Autodesk Inventor part; units mm, degrees
(part 3 of 4)
  circle A565 centre (25.95, -42.62) radius 1.125 construction
  circle A566 centre (31.03, -42.62) radius 1.125 construction
  circle A567 centre (36.11, -42.62) radius 1.125 construction
  circle A568 centre (41.19, -42.62) radius 1.125 construction
  circle A569 centre (46.27, -42.62) radius 1.125 construction
  circle A570 centre (51.35, -42.62) radius 1.125 construction
  circle A571 centre (56.43, -42.62) radius 1.125 construction
  circle A572 centre (61.51, -42.62) radius 1.125 construction
  circle A573 centre (66.59, -42.62) radius 1.125 construction
  circle A574 centre (71.67, -42.62) radius 1.125 construction
  circle A575 centre (76.75, -42.62) radius 1.125 construction
  circle A576 centre (81.83, -42.62) radius 1.125 construction
  circle A577 centre (10.71, -40.08) radius 1.125 construction
  circle A578 centre (15.79, -40.08) radius 1.125 construction
  circle A579 centre (20.87, -40.08) radius 1.125 construction
  circle A580 centre (25.95, -40.08) radius 1.125 construction
  circle A581 centre (31.03, -40.08) radius 1.125 construction
  circle A582 centre (36.11, -40.08) radius 1.125 construction
  circle A583 centre (41.19, -40.08) radius 1.125 construction
  circle A584 centre (46.27, -40.08) radius 1.125 construction
  circle A585 centre (51.35, -40.08) radius 1.125 construction
  circle A586 centre (56.43, -40.08) radius 1.125 construction
  circle A587 centre (61.51, -40.08) radius 1.125 construction
  circle A588 centre (66.59, -40.08) radius 1.125 construction
  circle A589 centre (71.67, -40.08) radius 1.125 construction
  circle A590 centre (76.75, -40.08) radius 1.125 construction
  circle A591 centre (81.83, -40.08) radius 1.125 construction
  circle A592 centre (10.71, -37.54) radius 1.125 construction
  circle A593 centre (15.79, -37.54) radius 1.125 construction
  circle A594 centre (20.87, -37.54) radius 1.125 construction
  circle A595 centre (25.95, -37.54) radius 1.125 construction
  circle A596 centre (31.03, -37.54) radius 1.125 construction
  circle A597 centre (36.11, -37.54) radius 1.125 construction
  circle A598 centre (41.19, -37.54) radius 1.125 construction
  circle A599 centre (46.27, -37.54) radius 1.125 construction
  circle A600 centre (51.35, -37.54) radius 1.125 construction
  circle A601 centre (56.43, -37.54) radius 1.125 construction
  circle A602 centre (61.51, -37.54) radius 1.125 construction
  circle A603 centre (66.59, -37.54) radius 1.125 construction
  circle A604 centre (71.67, -37.54) radius 1.125 construction
  circle A605 centre (76.75, -37.54) radius 1.125 construction
  circle A606 centre (81.83, -37.54) radius 1.125 construction
  circle A607 centre (10.71, -35) radius 1.125 construction
  circle A608 centre (15.79, -35) radius 1.125 construction
  circle A609 centre (20.87, -35) radius 1.125 construction
  circle A610 centre (25.95, -35) radius 1.125 construction
  circle A611 centre (31.03, -35) radius 1.125 construction
  circle A612 centre (36.11, -35) radius 1.125 construction
  circle A613 centre (41.19, -35) radius 1.125 construction
  circle A614 centre (46.27, -35) radius 1.125 construction
  circle A615 centre (51.35, -35) radius 1.125 construction
  circle A616 centre (56.43, -35) radius 1.125 construction
  circle A617 centre (61.51, -35) radius 1.125 construction
  circle A618 centre (66.59, -35) radius 1.125 construction
  circle A619 centre (71.67, -35) radius 1.125 construction
  circle A620 centre (76.75, -35) radius 1.125 construction
  circle A621 centre (81.83, -35) radius 1.125 construction
  circle A622 centre (10.71, -32.46) radius 1.125 construction
  circle A623 centre (15.79, -32.46) radius 1.125 construction
  circle A624 centre (20.87, -32.46) radius 1.125 construction
  circle A625 centre (25.95, -32.46) radius 1.125 construction
  circle A626 centre (31.03, -32.46) radius 1.125 construction
  circle A627 centre (36.11, -32.46) radius 1.125 construction
  circle A628 centre (41.19, -32.46) radius 1.125 construction
  circle A629 centre (46.27, -32.46) radius 1.125 construction
  circle A630 centre (51.35, -32.46) radius 1.125 construction
  circle A631 centre (56.43, -32.46) radius 1.125 construction
  circle A632 centre (61.51, -32.46) radius 1.125 construction
  circle A633 centre (66.59, -32.46) radius 1.125 construction
  circle A634 centre (71.67, -32.46) radius 1.125 construction
  circle A635 centre (76.75, -32.46) radius 1.125 construction
  circle A636 centre (81.83, -32.46) radius 1.125 construction
  circle A637 centre (10.71, -29.92) radius 1.125 construction
  circle A638 centre (15.79, -29.92) radius 1.125 construction
  circle A639 centre (20.87, -29.92) radius 1.125 construction
  circle A640 centre (25.95, -29.92) radius 1.125 construction
  circle A641 centre (31.03, -29.92) radius 1.125 construction
  circle A642 centre (36.11, -29.92) radius 1.125 construction
  circle A643 centre (41.19, -29.92) radius 1.125 construction
  circle A644 centre (46.27, -29.92) radius 1.125 construction
  circle A645 centre (51.35, -29.92) radius 1.125 construction
  circle A646 centre (56.43, -29.92) radius 1.125 construction
  circle A647 centre (61.51, -29.92) radius 1.125 construction
  circle A648 centre (66.59, -29.92) radius 1.125 construction
  circle A649 centre (71.67, -29.92) radius 1.125 construction
  circle A650 centre (76.75, -29.92) radius 1.125 construction
  circle A651 centre (81.83, -29.92) radius 1.125 construction
  circle A652 centre (10.71, -27.38) radius 1.125 construction
  circle A653 centre (15.79, -27.38) radius 1.125 construction
  circle A654 centre (20.87, -27.38) radius 1.125 construction
  circle A655 centre (25.95, -27.38) radius 1.125 construction
  circle A656 centre (31.03, -27.38) radius 1.125 construction
  circle A657 centre (36.11, -27.38) radius 1.125 construction
  circle A658 centre (41.19, -27.38) radius 1.125 construction
  circle A659 centre (46.27, -27.38) radius 1.125 construction
  circle A660 centre (51.35, -27.38) radius 1.125 construction
  circle A661 centre (56.43, -27.38) radius 1.125 construction
  circle A662 centre (61.51, -27.38) radius 1.125 construction
  circle A663 centre (66.59, -27.38) radius 1.125 construction
  circle A664 centre (71.67, -27.38) radius 1.125 construction
  circle A665 centre (76.75, -27.38) radius 1.125 construction
  circle A666 centre (81.83, -27.38) radius 1.125 construction
  circle A667 centre (10.71, -24.84) radius 1.125 construction
  circle A668 centre (15.79, -24.84) radius 1.125 construction
  circle A669 centre (20.87, -24.84) radius 1.125 construction
  circle A670 centre (25.95, -24.84) radius 1.125 construction
  circle A671 centre (31.03, -24.84) radius 1.125 construction
  circle A672 centre (36.11, -24.84) radius 1.125 construction
  circle A673 centre (41.19, -24.84) radius 1.125 construction
  circle A674 centre (46.27, -24.84) radius 1.125 construction
  circle A675 centre (51.35, -24.84) radius 1.125 construction
  circle A676 centre (56.43, -24.84) radius 1.125 construction
  circle A677 centre (61.51, -24.84) radius 1.125 construction
  circle A678 centre (66.59, -24.84) radius 1.125 construction
  circle A679 centre (71.67, -24.84) radius 1.125 construction
  circle A680 centre (76.75, -24.84) radius 1.125 construction
  circle A681 centre (81.83, -24.84) radius 1.125 construction
  circle A682 centre (10.71, -22.3) radius 1.125 construction
  circle A683 centre (15.79, -22.3) radius 1.125 construction
  circle A684 centre (20.87, -22.3) radius 1.125 construction
  circle A685 centre (25.95, -22.3) radius 1.125 construction
  circle A686 centre (31.03, -22.3) radius 1.125 construction
  circle A687 centre (36.11, -22.3) radius 1.125 construction
  circle A688 centre (41.19, -22.3) radius 1.125 construction
  circle A689 centre (46.27, -22.3) radius 1.125 construction
  circle A690 centre (51.35, -22.3) radius 1.125 construction
  circle A691 centre (56.43, -22.3) radius 1.125 construction
  circle A692 centre (61.51, -22.3) radius 1.125 construction
  circle A693 centre (66.59, -22.3) radius 1.125 construction
  circle A694 centre (71.67, -22.3) radius 1.125 construction
  circle A695 centre (76.75, -22.3) radius 1.125 construction
  circle A696 centre (81.83, -22.3) radius 1.125 construction
  circle A697 centre (10.71, -19.76) radius 1.125 construction
  circle A698 centre (15.79, -19.76) radius 1.125 construction
  circle A699 centre (20.87, -19.76) radius 1.125 construction
  circle A700 centre (25.95, -19.76) radius 1.125 construction
  circle A701 centre (31.03, -19.76) radius 1.125 construction
  circle A702 centre (36.11, -19.76) radius 1.125 construction
  circle A703 centre (41.19, -19.76) radius 1.125 construction
  circle A704 centre (46.27, -19.76) radius 1.125 construction
  circle A705 centre (51.35, -19.76) radius 1.125 construction
  circle A706 centre (56.43, -19.76) radius 1.125 construction
  circle A707 centre (61.51, -19.76) radius 1.125 construction
  circle A708 centre (66.59, -19.76) radius 1.125 construction
  circle A709 centre (71.67, -19.76) radius 1.125 construction
  circle A710 centre (76.75, -19.76) radius 1.125 construction
  circle A711 centre (81.83, -19.76) radius 1.125 construction
  circle A712 centre (10.71, -17.22) radius 1.125 construction
  circle A713 centre (15.79, -17.22) radius 1.125 construction
  circle A714 centre (20.87, -17.22) radius 1.125 construction
  circle A715 centre (25.95, -17.22) radius 1.125 construction
  circle A716 centre (31.03, -17.22) radius 1.125 construction
  circle A717 centre (36.11, -17.22) radius 1.125 construction
  circle A718 centre (41.19, -17.22) radius 1.125 construction
  circle A719 centre (46.27, -17.22) radius 1.125 construction
  circle A720 centre (51.35, -17.22) radius 1.125 construction
  circle A721 centre (56.43, -17.22) radius 1.125 construction
  circle A722 centre (61.51, -17.22) radius 1.125 construction
  circle A723 centre (66.59, -17.22) radius 1.125 construction
  circle A724 centre (71.67, -17.22) radius 1.125 construction
  circle A725 centre (76.75, -17.22) radius 1.125 construction
  circle A726 centre (81.83, -17.22) radius 1.125 construction
  circle A727 centre (10.71, -14.68) radius 1.125 construction
  circle A728 centre (15.79, -14.68) radius 1.125 construction
  circle A729 centre (20.87, -14.68) radius 1.125 construction
  circle A730 centre (25.95, -14.68) radius 1.125 construction
  circle A731 centre (31.03, -14.68) radius 1.125 construction
  circle A732 centre (36.11, -14.68) radius 1.125 construction
  circle A733 centre (41.19, -14.68) radius 1.125 construction
  circle A734 centre (46.27, -14.68) radius 1.125 construction
  circle A735 centre (51.35, -14.68) radius 1.125 construction
  circle A736 centre (56.43, -14.68) radius 1.125 construction
  circle A737 centre (61.51, -14.68) radius 1.125 construction
  circle A738 centre (66.59, -14.68) radius 1.125 construction
  circle A739 centre (71.67, -14.68) radius 1.125 construction
  circle A740 centre (76.75, -14.68) radius 1.125 construction
  circle A741 centre (81.83, -14.68) radius 1.125 construction
  circle A742 centre (10.71, -12.14) radius 1.125 construction
  circle A743 centre (15.79, -12.14) radius 1.125 construction
  circle A744 centre (20.87, -12.14) radius 1.125 construction
  circle A745 centre (25.95, -12.14) radius 1.125 construction
  circle A746 centre (31.03, -12.14) radius 1.125 construction
  circle A747 centre (36.11, -12.14) radius 1.125 construction
  circle A748 centre (41.19, -12.14) radius 1.125 construction
  circle A749 centre (46.27, -12.14) radius 1.125 construction
  circle A750 centre (51.35, -12.14) radius 1.125 construction
  circle A751 centre (56.43, -12.14) radius 1.125 construction
  circle A752 centre (61.51, -12.14) radius 1.125 construction
  circle A753 centre (66.59, -12.14) radius 1.125 construction
  circle A754 centre (71.67, -12.14) radius 1.125 construction
  circle A755 centre (76.75, -12.14) radius 1.125 construction
  circle A756 centre (81.83, -12.14) radius 1.125 construction
  circle A757 centre (10.71, -9.6) radius 1.125 construction
  circle A758 centre (15.79, -9.6) radius 1.125 construction
  circle A759 centre (20.87, -9.6) radius 1.125 construction
  circle A760 centre (25.95, -9.6) radius 1.125 construction
  circle A761 centre (31.03, -9.6) radius 1.125 construction
  circle A762 centre (36.11, -9.6) radius 1.125 construction
  circle A763 centre (41.19, -9.6) radius 1.125 construction
  circle A764 centre (46.27, -9.6) radius 1.125 construction
  circle A765 centre (51.35, -9.6) radius 1.125 construction
  circle A766 centre (56.43, -9.6) radius 1.125 construction
  circle A767 centre (61.51, -9.6) radius 1.125 construction
  circle A768 centre (66.59, -9.6) radius 1.125 construction
  circle A769 centre (71.67, -9.6) radius 1.125 construction
  circle A770 centre (76.75, -9.6) radius 1.125 construction
  circle A771 centre (81.83, -9.6) radius 1.125 construction
  circle A772 centre (10.71, -7.06) radius 1.125 construction
  circle A773 centre (15.79, -7.06) radius 1.125 construction
  circle A774 centre (20.87, -7.06) radius 1.125 construction
  circle A775 centre (25.95, -7.06) radius 1.125 construction
  circle A776 centre (31.03, -7.06) radius 1.125 construction
  circle A777 centre (36.11, -7.06) radius 1.125 construction
  circle A778 centre (41.19, -7.06) radius 1.125 construction
  circle A779 centre (46.27, -7.06) radius 1.125 construction
  circle A780 centre (51.35, -7.06) radius 1.125 construction
  circle A781 centre (56.43, -7.06) radius 1.125 construction
  circle A782 centre (61.51, -7.06) radius 1.125 construction
  circle A783 centre (66.59, -7.06) radius 1.125 construction
  circle A784 centre (71.67, -7.06) radius 1.125 construction
  circle A785 centre (76.75, -7.06) radius 1.125 construction
  circle A786 centre (81.83, -7.06) radius 1.125 construction
  circle A787 centre (10.71, -4.52) radius 1.125 construction
  circle A788 centre (15.79, -4.52) radius 1.125 construction
  circle A789 centre (20.87, -4.52) radius 1.125 construction
  circle A790 centre (25.95, -4.52) radius 1.125 construction
  circle A791 centre (31.03, -4.52) radius 1.125 construction
  circle A792 centre (36.11, -4.52) radius 1.125 construction
  circle A793 centre (41.19, -4.52) radius 1.125 construction
  circle A794 centre (46.27, -4.52) radius 1.125 construction
  circle A795 centre (51.35, -4.52) radius 1.125 construction
  circle A796 centre (56.43, -4.52) radius 1.125 construction
  circle A797 centre (61.51, -4.52) radius 1.125 construction
  circle A798 centre (66.59, -4.52) radius 1.125 construction
  circle A799 centre (71.67, -4.52) radius 1.125 construction
  circle A800 centre (76.75, -4.52) radius 1.125 construction
  circle A801 centre (81.83, -4.52) radius 1.125 construction
  circle A802 centre (4.36, -4.52) radius 1.5494 construction
  circle A803 centre (4.36, -65.48) radius 1.5494 construction
  circle A804 centre (85.64, -65.48) radius 1.5494 construction
  circle A805 centre (85.64, -4.52) radius 1.5494 construction
  line L52 (0, 0) -> (90, 0) construction
  line L53 (90, 0) -> (90, -70) construction
  line L54 (90, -70) -> (0, -70) construction
  line L55 (0, -70) -> (0, 0) construction
  circle A806 centre (8.17, -4.52) radius 0.625
  circle A807 centre (10.71, -4.52) radius 0.625
  circle A808 centre (13.25, -4.52) radius 0.625
  circle A809 centre (15.79, -4.52) radius 0.625
  circle A810 centre (18.33, -4.52) radius 0.625
  circle A811 centre (20.87, -4.52) radius 0.625
  circle A812 centre (23.41, -4.52) radius 0.625
  circle A813 centre (25.95, -4.52) radius 0.625
  circle A814 centre (28.49, -4.52) radius 0.625
  circle A815 centre (31.03, -4.52) radius 0.625
  circle A816 centre (33.57, -4.52) radius 0.625
  circle A817 centre (36.11, -4.52) radius 0.625
  circle A818 centre (38.65, -4.52) radius 0.625
  circle A819 centre (41.19, -4.52) radius 0.625
  circle A820 centre (43.73, -4.52) radius 0.625
  circle A821 centre (46.27, -4.52) radius 0.625
  circle A822 centre (48.81, -4.52) radius 0.625
  circle A823 centre (51.35, -4.52) radius 0.625
  circle A824 centre (53.89, -4.52) radius 0.625
  circle A825 centre (56.43, -4.52) radius 0.625
  circle A826 centre (58.97, -4.52) radius 0.625
  circle A827 centre (61.51, -4.52) radius 0.625
  circle A828 centre (64.05, -4.52) radius 0.625
  circle A829 centre (66.59, -4.52) radius 0.625
  circle A830 centre (69.13, -4.52) radius 0.625
  circle A831 centre (71.67, -4.52) radius 0.625
  circle A832 centre (74.21, -4.52) radius 0.625
  circle A833 centre (76.75, -4.52) radius 0.625
  circle A834 centre (79.29, -4.52) radius 0.625
  circle A835 centre (81.83, -4.52) radius 0.625
  circle A836 centre (8.17, -7.06) radius 0.625
  circle A837 centre (10.71, -7.06) radius 0.625
  circle A838 centre (13.25, -7.06) radius 0.625
  circle A839 centre (15.79, -7.06) radius 0.625
  circle A840 centre (18.33, -7.06) radius 0.625
  circle A841 centre (20.87, -7.06) radius 0.625
  circle A842 centre (23.41, -7.06) radius 0.625
  circle A843 centre (25.95, -7.06) radius 0.625
  circle A844 centre (28.49, -7.06) radius 0.625
  circle A845 centre (31.03, -7.06) radius 0.625
  circle A846 centre (33.57, -7.06) radius 0.625
  circle A847 centre (36.11, -7.06) radius 0.625
  circle A848 centre (38.65, -7.06) radius 0.625
  circle A849 centre (41.19, -7.06) radius 0.625
  circle A850 centre (43.73, -7.06) radius 0.625
  circle A851 centre (46.27, -7.06) radius 0.625
  circle A852 centre (48.81, -7.06) radius 0.625
  circle A853 centre (51.35, -7.06) radius 0.625
  circle A854 centre (53.89, -7.06) radius 0.625
  circle A855 centre (56.43, -7.06) radius 0.625
  circle A856 centre (58.97, -7.06) radius 0.625
  circle A857 centre (61.51, -7.06) radius 0.625
  circle A858 centre (64.05, -7.06) radius 0.625
  circle A859 centre (66.59, -7.06) radius 0.625
  circle A860 centre (69.13, -7.06) radius 0.625
  circle A861 centre (71.67, -7.06) radius 0.625
  circle A862 centre (74.21, -7.06) radius 0.625
  circle A863 centre (76.75, -7.06) radius 0.625
  circle A864 centre (79.29, -7.06) radius 0.625
  circle A865 centre (81.83, -7.06) radius 0.625
  circle A866 centre (8.17, -9.6) radius 0.625
  circle A867 centre (10.71, -9.6) radius 0.625
  circle A868 centre (13.25, -9.6) radius 0.625
  circle A869 centre (15.79, -9.6) radius 0.625
  circle A870 centre (18.33, -9.6) radius 0.625
  circle A871 centre (20.87, -9.6) radius 0.625
  circle A872 centre (23.41, -9.6) radius 0.625
  circle A873 centre (25.95, -9.6) radius 0.625
  circle A874 centre (28.49, -9.6) radius 0.625
  circle A875 centre (31.03, -9.6) radius 0.625
  circle A876 centre (33.57, -9.6) radius 0.625
  circle A877 centre (36.11, -9.6) radius 0.625
  circle A878 centre (38.65, -9.6) radius 0.625
  circle A879 centre (41.19, -9.6) radius 0.625
  circle A880 centre (43.73, -9.6) radius 0.625
  circle A881 centre (46.27, -9.6) radius 0.625
  circle A882 centre (48.81, -9.6) radius 0.625
  circle A883 centre (51.35, -9.6) radius 0.625
  circle A884 centre (53.89, -9.6) radius 0.625
  circle A885 centre (56.43, -9.6) radius 0.625
  circle A886 centre (58.97, -9.6) radius 0.625
  circle A887 centre (61.51, -9.6) radius 0.625
  circle A888 centre (64.05, -9.6) radius 0.625
  circle A889 centre (66.59, -9.6) radius 0.625
  circle A890 centre (69.13, -9.6) radius 0.625
  circle A891 centre (71.67, -9.6) radius 0.625
  circle A892 centre (74.21, -9.6) radius 0.625
  circle A893 centre (76.75, -9.6) radius 0.625
  circle A894 centre (79.29, -9.6) radius 0.625
  circle A895 centre (81.83, -9.6) radius 0.625
  circle A896 centre (8.17, -12.14) radius 0.625
  circle A897 centre (10.71, -12.14) radius 0.625
  circle A898 centre (13.25, -12.14) radius 0.625
  circle A899 centre (15.79, -12.14) radius 0.625
  circle A900 centre (18.33, -12.14) radius 0.625
  circle A901 centre (20.87, -12.14) radius 0.625
  circle A902 centre (23.41, -12.14) radius 0.625
  circle A903 centre (25.95, -12.14) radius 0.625
  circle A904 centre (28.49, -12.14) radius 0.625
  circle A905 centre (31.03, -12.14) radius 0.625
  circle A906 centre (33.57, -12.14) radius 0.625
  circle A907 centre (36.11, -12.14) radius 0.625
  circle A908 centre (38.65, -12.14) radius 0.625
  circle A909 centre (41.19, -12.14) radius 0.625
  circle A910 centre (43.73, -12.14) radius 0.625
  circle A911 centre (46.27, -12.14) radius 0.625
  circle A912 centre (48.81, -12.14) radius 0.625
  circle A913 centre (51.35, -12.14) radius 0.625
  circle A914 centre (53.89, -12.14) radius 0.625
  circle A915 centre (56.43, -12.14) radius 0.625
  circle A916 centre (58.97, -12.14) radius 0.625
  circle A917 centre (61.51, -12.14) radius 0.625
  circle A918 centre (64.05, -12.14) radius 0.625
  circle A919 centre (66.59, -12.14) radius 0.625
  circle A920 centre (69.13, -12.14) radius 0.625
  circle A921 centre (71.67, -12.14) radius 0.625
  circle A922 centre (74.21, -12.14) radius 0.625
  circle A923 centre (76.75, -12.14) radius 0.625
  circle A924 centre (79.29, -12.14) radius 0.625
  circle A925 centre (81.83, -12.14) radius 0.625
  circle A926 centre (8.17, -14.68) radius 0.625
  circle A927 centre (10.71, -14.68) radius 0.625
  circle A928 centre (13.25, -14.68) radius 0.625
  circle A929 centre (15.79, -14.68) radius 0.625
  circle A930 centre (18.33, -14.68) radius 0.625
  circle A931 centre (20.87, -14.68) radius 0.625
  circle A932 centre (23.41, -14.68) radius 0.625
  circle A933 centre (25.95, -14.68) radius 0.625
  circle A934 centre (28.49, -14.68) radius 0.625
  circle A935 centre (31.03, -14.68) radius 0.625
  circle A936 centre (33.57, -14.68) radius 0.625
  circle A937 centre (36.11, -14.68) radius 0.625
  circle A938 centre (38.65, -14.68) radius 0.625
  circle A939 centre (41.19, -14.68) radius 0.625
  circle A940 centre (43.73, -14.68) radius 0.625
  circle A941 centre (46.27, -14.68) radius 0.625
  circle A942 centre (48.81, -14.68) radius 0.625
  circle A943 centre (51.35, -14.68) radius 0.625
  circle A944 centre (53.89, -14.68) radius 0.625
  circle A945 centre (56.43, -14.68) radius 0.625
  circle A946 centre (58.97, -14.68) radius 0.625
  circle A947 centre (61.51, -14.68) radius 0.625
  circle A948 centre (64.05, -14.68) radius 0.625
  circle A949 centre (66.59, -14.68) radius 0.625
  circle A950 centre (69.13, -14.68) radius 0.625
  circle A951 centre (71.67, -14.68) radius 0.625
  circle A952 centre (74.21, -14.68) radius 0.625
  circle A953 centre (76.75, -14.68) radius 0.625
  circle A954 centre (79.29, -14.68) radius 0.625
  circle A955 centre (81.83, -14.68) radius 0.625
  circle A956 centre (8.17, -17.22) radius 0.625
  circle A957 centre (10.71, -17.22) radius 0.625
  circle A958 centre (13.25, -17.22) radius 0.625
  circle A959 centre (15.79, -17.22) radius 0.625
  circle A960 centre (18.33, -17.22) radius 0.625
  circle A961 centre (20.87, -17.22) radius 0.625
  circle A962 centre (23.41, -17.22) radius 0.625
  circle A963 centre (25.95, -17.22) radius 0.625
  circle A964 centre (28.49, -17.22) radius 0.625
  circle A965 centre (31.03, -17.22) radius 0.625
  circle A966 centre (33.57, -17.22) radius 0.625
  circle A967 centre (36.11, -17.22) radius 0.625
  circle A968 centre (38.65, -17.22) radius 0.625
  circle A969 centre (41.19, -17.22) radius 0.625
  circle A970 centre (43.73, -17.22) radius 0.625
  circle A971 centre (46.27, -17.22) radius 0.625
  circle A972 centre (48.81, -17.22) radius 0.625
  circle A973 centre (51.35, -17.22) radius 0.625
  circle A974 centre (53.89, -17.22) radius 0.625
  circle A975 centre (56.43, -17.22) radius 0.625
  circle A976 centre (58.97, -17.22) radius 0.625
  circle A977 centre (61.51, -17.22) radius 0.625
  circle A978 centre (64.05, -17.22) radius 0.625
  circle A979 centre (66.59, -17.22) radius 0.625
  circle A980 centre (69.13, -17.22) radius 0.625
  circle A981 centre (71.67, -17.22) radius 0.625
  circle A982 centre (74.21, -17.22) radius 0.625
  circle A983 centre (76.75, -17.22) radius 0.625
  circle A984 centre (79.29, -17.22) radius 0.625
  circle A985 centre (81.83, -17.22) radius 0.625
  circle A986 centre (8.17, -19.76) radius 0.625
  circle A987 centre (10.71, -19.76) radius 0.625
  circle A988 centre (13.25, -19.76) radius 0.625
  circle A989 centre (15.79, -19.76) radius 0.625
  circle A990 centre (18.33, -19.76) radius 0.625
  circle A991 centre (20.87, -19.76) radius 0.625
  circle A992 centre (23.41, -19.76) radius 0.625
  circle A993 centre (25.95, -19.76) radius 0.625
  circle A994 centre (28.49, -19.76) radius 0.625
  circle A995 centre (31.03, -19.76) radius 0.625
  circle A996 centre (33.57, -19.76) radius 0.625
  circle A997 centre (36.11, -19.76) radius 0.625
  circle A998 centre (38.65, -19.76) radius 0.625
  circle A999 centre (41.19, -19.76) radius 0.625
  circle A1000 centre (43.73, -19.76) radius 0.625
  circle A1001 centre (46.27, -19.76) radius 0.625
  circle A1002 centre (48.81, -19.76) radius 0.625
  circle A1003 centre (51.35, -19.76) radius 0.625
  circle A1004 centre (53.89, -19.76) radius 0.625
  circle A1005 centre (56.43, -19.76) radius 0.625
  circle A1006 centre (58.97, -19.76) radius 0.625
  circle A1007 centre (61.51, -19.76) radius 0.625
  circle A1008 centre (64.05, -19.76) radius 0.625
  circle A1009 centre (66.59, -19.76) radius 0.625
  circle A1010 centre (69.13, -19.76) radius 0.625
  circle A1011 centre (71.67, -19.76) radius 0.625
  circle A1012 centre (74.21, -19.76) radius 0.625
  circle A1013 centre (76.75, -19.76) radius 0.625
  circle A1014 centre (79.29, -19.76) radius 0.625
  circle A1015 centre (81.83, -19.76) radius 0.625
  circle A1016 centre (8.17, -22.3) radius 0.625
  circle A1017 centre (10.71, -22.3) radius 0.625
  circle A1018 centre (13.25, -22.3) radius 0.625
  circle A1019 centre (15.79, -22.3) radius 0.625
  circle A1020 centre (18.33, -22.3) radius 0.625
  circle A1021 centre (20.87, -22.3) radius 0.625
  circle A1022 centre (23.41, -22.3) radius 0.625
  circle A1023 centre (25.95, -22.3) radius 0.625
  circle A1024 centre (28.49, -22.3) radius 0.625
  circle A1025 centre (31.03, -22.3) radius 0.625
  circle A1026 centre (33.57, -22.3) radius 0.625
  circle A1027 centre (36.11, -22.3) radius 0.625
  circle A1028 centre (38.65, -22.3) radius 0.625
  circle A1029 centre (41.19, -22.3) radius 0.625
  circle A1030 centre (43.73, -22.3) radius 0.625
  circle A1031 centre (46.27, -22.3) radius 0.625
  circle A1032 centre (48.81, -22.3) radius 0.625
  circle A1033 centre (51.35, -22.3) radius 0.625
  circle A1034 centre (53.89, -22.3) radius 0.625
  circle A1035 centre (56.43, -22.3) radius 0.625
  circle A1036 centre (58.97, -22.3) radius 0.625
  circle A1037 centre (61.51, -22.3) radius 0.625
  circle A1038 centre (64.05, -22.3) radius 0.625
  circle A1039 centre (66.59, -22.3) radius 0.625
  circle A1040 centre (69.13, -22.3) radius 0.625
  circle A1041 centre (71.67, -22.3) radius 0.625
  circle A1042 centre (74.21, -22.3) radius 0.625
  circle A1043 centre (76.75, -22.3) radius 0.625
  circle A1044 centre (79.29, -22.3) radius 0.625
  circle A1045 centre (81.83, -22.3) radius 0.625
  circle A1046 centre (8.17, -24.84) radius 0.625
  circle A1047 centre (10.71, -24.84) radius 0.625
  circle A1048 centre (13.25, -24.84) radius 0.625
  circle A1049 centre (15.79, -24.84) radius 0.625
  circle A1050 centre (18.33, -24.84) radius 0.625
  circle A1051 centre (20.87, -24.84) radius 0.625
  circle A1052 centre (23.41, -24.84) radius 0.625
  circle A1053 centre (25.95, -24.84) radius 0.625
  circle A1054 centre (28.49, -24.84) radius 0.625
  circle A1055 centre (31.03, -24.84) radius 0.625
  circle A1056 centre (33.57, -24.84) radius 0.625
  circle A1057 centre (36.11, -24.84) radius 0.625
  circle A1058 centre (38.65, -24.84) radius 0.625
  circle A1059 centre (41.19, -24.84) radius 0.625
  circle A1060 centre (43.73, -24.84) radius 0.625
  circle A1061 centre (46.27, -24.84) radius 0.625
  circle A1062 centre (48.81, -24.84) radius 0.625
  circle A1063 centre (51.35, -24.84) radius 0.625
  circle A1064 centre (53.89, -24.84) radius 0.625
  circle A1065 centre (56.43, -24.84) radius 0.625
  circle A1066 centre (58.97, -24.84) radius 0.625
  circle A1067 centre (61.51, -24.84) radius 0.625
  circle A1068 centre (64.05, -24.84) radius 0.625
  circle A1069 centre (66.59, -24.84) radius 0.625
  circle A1070 centre (69.13, -24.84) radius 0.625
  circle A1071 centre (71.67, -24.84) radius 0.625
  circle A1072 centre (74.21, -24.84) radius 0.625
  circle A1073 centre (76.75, -24.84) radius 0.625
  circle A1074 centre (79.29, -24.84) radius 0.625
  circle A1075 centre (81.83, -24.84) radius 0.625
  circle A1076 centre (8.17, -27.38) radius 0.625
  circle A1077 centre (10.71, -27.38) radius 0.625
  circle A1078 centre (13.25, -27.38) radius 0.625
  circle A1079 centre (15.79, -27.38) radius 0.625
  circle A1080 centre (18.33, -27.38) radius 0.625
  circle A1081 centre (20.87, -27.38) radius 0.625
  circle A1082 centre (23.41, -27.38) radius 0.625
  circle A1083 centre (25.95, -27.38) radius 0.625
  circle A1084 centre (28.49, -27.38) radius 0.625
  circle A1085 centre (31.03, -27.38) radius 0.625
  circle A1086 centre (33.57, -27.38) radius 0.625
  circle A1087 centre (36.11, -27.38) radius 0.625
  circle A1088 centre (38.65, -27.38) radius 0.625
  circle A1089 centre (41.19, -27.38) radius 0.625
  circle A1090 centre (43.73, -27.38) radius 0.625
  circle A1091 centre (46.27, -27.38) radius 0.625
  circle A1092 centre (48.81, -27.38) radius 0.625
  circle A1093 centre (51.35, -27.38) radius 0.625
  circle A1094 centre (53.89, -27.38) radius 0.625
  circle A1095 centre (56.43, -27.38) radius 0.625
  circle A1096 centre (58.97, -27.38) radius 0.625
  circle A1097 centre (61.51, -27.38) radius 0.625
  circle A1098 centre (64.05, -27.38) radius 0.625
  circle A1099 centre (66.59, -27.38) radius 0.625
  circle A1100 centre (69.13, -27.38) radius 0.625
  circle A1101 centre (71.67, -27.38) radius 0.625
  circle A1102 centre (74.21, -27.38) radius 0.625
  circle A1103 centre (76.75, -27.38) radius 0.625
  circle A1104 centre (79.29, -27.38) radius 0.625
  circle A1105 centre (81.83, -27.38) radius 0.625
  circle A1106 centre (8.17, -29.92) radius 0.625
  circle A1107 centre (10.71, -29.92) radius 0.625
  circle A1108 centre (13.25, -29.92) radius 0.625
  circle A1109 centre (15.79, -29.92) radius 0.625
  circle A1110 centre (18.33, -29.92) radius 0.625
  circle A1111 centre (20.87, -29.92) radius 0.625
  circle A1112 centre (23.41, -29.92) radius 0.625
  circle A1113 centre (25.95, -29.92) radius 0.625
  circle A1114 centre (28.49, -29.92) radius 0.625
  circle A1115 centre (31.03, -29.92) radius 0.625
  circle A1116 centre (33.57, -29.92) radius 0.625
  circle A1117 centre (36.11, -29.92) radius 0.625
  circle A1118 centre (38.65, -29.92) radius 0.625
  circle A1119 centre (41.19, -29.92) radius 0.625
  circle A1120 centre (43.73, -29.92) radius 0.625
  circle A1121 centre (46.27, -29.92) radius 0.625
  circle A1122 centre (48.81, -29.92) radius 0.625
  circle A1123 centre (51.35, -29.92) radius 0.625
  circle A1124 centre (53.89, -29.92) radius 0.625
  circle A1125 centre (56.43, -29.92) radius 0.625
  circle A1126 centre (58.97, -29.92) radius 0.625
  circle A1127 centre (61.51, -29.92) radius 0.625
  circle A1128 centre (64.05, -29.92) radius 0.625
  circle A1129 centre (66.59, -29.92) radius 0.625
  circle A1130 centre (69.13, -29.92) radius 0.625
  circle A1131 centre (71.67, -29.92) radius 0.625
  circle A1132 centre (74.21, -29.92) radius 0.625
  circle A1133 centre (76.75, -29.92) radius 0.625
  circle A1134 centre (79.29, -29.92) radius 0.625
  circle A1135 centre (81.83, -29.92) radius 0.625
  circle A1136 centre (8.17, -32.46) radius 0.625
  circle A1137 centre (10.71, -32.46) radius 0.625
  circle A1138 centre (13.25, -32.46) radius 0.625
  circle A1139 centre (15.79, -32.46) radius 0.625
  circle A1140 centre (18.33, -32.46) radius 0.625
  circle A1141 centre (20.87, -32.46) radius 0.625
  circle A1142 centre (23.41, -32.46) radius 0.625
  circle A1143 centre (25.95, -32.46) radius 0.625
  circle A1144 centre (28.49, -32.46) radius 0.625
  circle A1145 centre (31.03, -32.46) radius 0.625
  circle A1146 centre (33.57, -32.46) radius 0.625
  circle A1147 centre (36.11, -32.46) radius 0.625
  circle A1148 centre (38.65, -32.46) radius 0.625
  circle A1149 centre (41.19, -32.46) radius 0.625
  circle A1150 centre (43.73, -32.46) radius 0.625
  circle A1151 centre (46.27, -32.46) radius 0.625
  circle A1152 centre (48.81, -32.46) radius 0.625
  circle A1153 centre (51.35, -32.46) radius 0.625
  circle A1154 centre (53.89, -32.46) radius 0.625
  circle A1155 centre (56.43, -32.46) radius 0.625
  circle A1156 centre (58.97, -32.46) radius 0.625
  circle A1157 centre (61.51, -32.46) radius 0.625
  circle A1158 centre (64.05, -32.46) radius 0.625
  circle A1159 centre (66.59, -32.46) radius 0.625
  circle A1160 centre (69.13, -32.46) radius 0.625
  circle A1161 centre (71.67, -32.46) radius 0.625
  circle A1162 centre (74.21, -32.46) radius 0.625
  circle A1163 centre (76.75, -32.46) radius 0.625
  circle A1164 centre (79.29, -32.46) radius 0.625
  circle A1165 centre (81.83, -32.46) radius 0.625
  circle A1166 centre (8.17, -35) radius 0.625
  circle A1167 centre (10.71, -35) radius 0.625
  circle A1168 centre (13.25, -35) radius 0.625
  circle A1169 centre (15.79, -35) radius 0.625
  circle A1170 centre (18.33, -35) radius 0.625
  circle A1171 centre (20.87, -35) radius 0.625
  circle A1172 centre (23.41, -35) radius 0.625
  circle A1173 centre (25.95, -35) radius 0.625
  circle A1174 centre (28.49, -35) radius 0.625
  circle A1175 centre (31.03, -35) radius 0.625
  circle A1176 centre (33.57, -35) radius 0.625
  circle A1177 centre (36.11, -35) radius 0.625
  circle A1178 centre (38.65, -35) radius 0.625
  circle A1179 centre (41.19, -35) radius 0.625
  circle A1180 centre (43.73, -35) radius 0.625
  circle A1181 centre (46.27, -35) radius 0.625
  circle A1182 centre (48.81, -35) radius 0.625
  circle A1183 centre (51.35, -35) radius 0.625
  circle A1184 centre (53.89, -35) radius 0.625
  circle A1185 centre (56.43, -35) radius 0.625
  circle A1186 centre (58.97, -35) radius 0.625
  circle A1187 centre (61.51, -35) radius 0.625
  circle A1188 centre (64.05, -35) radius 0.625
  circle A1189 centre (66.59, -35) radius 0.625
  circle A1190 centre (69.13, -35) radius 0.625
  circle A1191 centre (71.67, -35) radius 0.625
  circle A1192 centre (74.21, -35) radius 0.625
  circle A1193 centre (76.75, -35) radius 0.625
  circle A1194 centre (79.29, -35) radius 0.625
  circle A1195 centre (81.83, -35) radius 0.625
  circle A1196 centre (8.17, -37.54) radius 0.625
  circle A1197 centre (10.71, -37.54) radius 0.625
  circle A1198 centre (13.25, -37.54) radius 0.625
  circle A1199 centre (15.79, -37.54) radius 0.625
  circle A1200 centre (18.33, -37.54) radius 0.625
  circle A1201 centre (20.87, -37.54) radius 0.625
  circle A1202 centre (23.41, -37.54) radius 0.625
  circle A1203 centre (25.95, -37.54) radius 0.625
  circle A1204 centre (28.49, -37.54) radius 0.625
  circle A1205 centre (31.03, -37.54) radius 0.625
  circle A1206 centre (33.57, -37.54) radius 0.625
  circle A1207 centre (36.11, -37.54) radius 0.625
  circle A1208 centre (38.65, -37.54) radius 0.625
  circle A1209 centre (41.19, -37.54) radius 0.625
  circle A1210 centre (43.73, -37.54) radius 0.625
  circle A1211 centre (46.27, -37.54) radius 0.625
  circle A1212 centre (48.81, -37.54) radius 0.625
  circle A1213 centre (51.35, -37.54) radius 0.625
  circle A1214 centre (53.89, -37.54) radius 0.625
  circle A1215 centre (56.43, -37.54) radius 0.625
  circle A1216 centre (58.97, -37.54) radius 0.625
  circle A1217 centre (61.51, -37.54) radius 0.625
  circle A1218 centre (64.05, -37.54) radius 0.625
  circle A1219 centre (66.59, -37.54) radius 0.625
  circle A1220 centre (69.13, -37.54) radius 0.625
  circle A1221 centre (71.67, -37.54) radius 0.625
  circle A1222 centre (74.21, -37.54) radius 0.625
  circle A1223 centre (76.75, -37.54) radius 0.625
  circle A1224 centre (79.29, -37.54) radius 0.625
  circle A1225 centre (81.83, -37.54) radius 0.625
  circle A1226 centre (8.17, -40.08) radius 0.625
  circle A1227 centre (10.71, -40.08) radius 0.625
  circle A1228 centre (13.25, -40.08) radius 0.625
  circle A1229 centre (15.79, -40.08) radius 0.625
  circle A1230 centre (18.33, -40.08) radius 0.625
  circle A1231 centre (20.87, -40.08) radius 0.625
  circle A1232 centre (23.41, -40.08) radius 0.625
  circle A1233 centre (25.95, -40.08) radius 0.625
  circle A1234 centre (28.49, -40.08) radius 0.625
  circle A1235 centre (31.03, -40.08) radius 0.625
  circle A1236 centre (33.57, -40.08) radius 0.625
  circle A1237 centre (36.11, -40.08) radius 0.625
  circle A1238 centre (38.65, -40.08) radius 0.625
  circle A1239 centre (41.19, -40.08) radius 0.625
  circle A1240 centre (43.73, -40.08) radius 0.625
  circle A1241 centre (46.27, -40.08) radius 0.625
  circle A1242 centre (48.81, -40.08) radius 0.625
  circle A1243 centre (51.35, -40.08) radius 0.625
  circle A1244 centre (53.89, -40.08) radius 0.625
  circle A1245 centre (56.43, -40.08) radius 0.625
  circle A1246 centre (58.97, -40.08) radius 0.625
  circle A1247 centre (61.51, -40.08) radius 0.625
  circle A1248 centre (64.05, -40.08) radius 0.625
  circle A1249 centre (66.59, -40.08) radius 0.625
  circle A1250 centre (69.13, -40.08) radius 0.625
  circle A1251 centre (71.67, -40.08) radius 0.625
  circle A1252 centre (74.21, -40.08) radius 0.625
  circle A1253 centre (76.75, -40.08) radius 0.625
  circle A1254 centre (79.29, -40.08) radius 0.625
  circle A1255 centre (81.83, -40.08) radius 0.625
  circle A1256 centre (8.17, -42.62) radius 0.625
  circle A1257 centre (10.71, -42.62) radius 0.625
  circle A1258 centre (13.25, -42.62) radius 0.625
  circle A1259 centre (15.79, -42.62) radius 0.625
  circle A1260 centre (18.33, -42.62) radius 0.625
  circle A1261 centre (20.87, -42.62) radius 0.625
  circle A1262 centre (23.41, -42.62) radius 0.625
  circle A1263 centre (25.95, -42.62) radius 0.625
  circle A1264 centre (28.49, -42.62) radius 0.625
  circle A1265 centre (31.03, -42.62) radius 0.625
  circle A1266 centre (33.57, -42.62) radius 0.625
  circle A1267 centre (36.11, -42.62) radius 0.625
  circle A1268 centre (38.65, -42.62) radius 0.625
  circle A1269 centre (41.19, -42.62) radius 0.625
  circle A1270 centre (43.73, -42.62) radius 0.625
  circle A1271 centre (46.27, -42.62) radius 0.625
  circle A1272 centre (48.81, -42.62) radius 0.625
  circle A1273 centre (51.35, -42.62) radius 0.625
  circle A1274 centre (53.89, -42.62) radius 0.625
  circle A1275 centre (56.43, -42.62) radius 0.625
  circle A1276 centre (58.97, -42.62) radius 0.625
  circle A1277 centre (61.51, -42.62) radius 0.625
  circle A1278 centre (64.05, -42.62) radius 0.625
  circle A1279 centre (66.59, -42.62) radius 0.625
  circle A1280 centre (69.13, -42.62) radius 0.625
  circle A1281 centre (71.67, -42.62) radius 0.625
  circle A1282 centre (74.21, -42.62) radius 0.625
  circle A1283 centre (76.75, -42.62) radius 0.625
  circle A1284 centre (79.29, -42.62) radius 0.625
  circle A1285 centre (81.83, -42.62) radius 0.625
  circle A1286 centre (8.17, -45.16) radius 0.625
  circle A1287 centre (10.71, -45.16) radius 0.625
  circle A1288 centre (13.25, -45.16) radius 0.625
  circle A1289 centre (15.79, -45.16) radius 0.625
  circle A1290 centre (18.33, -45.16) radius 0.625
  circle A1291 centre (20.87, -45.16) radius 0.625
  circle A1292 centre (23.41, -45.16) radius 0.625
  circle A1293 centre (25.95, -45.16) radius 0.625
  circle A1294 centre (28.49, -45.16) radius 0.625
  circle A1295 centre (31.03, -45.16) radius 0.625
  circle A1296 centre (33.57, -45.16) radius 0.625
  circle A1297 centre (36.11, -45.16) radius 0.625
  circle A1298 centre (38.65, -45.16) radius 0.625
  circle A1299 centre (41.19, -45.16) radius 0.625
  circle A1300 centre (43.73, -45.16) radius 0.625
  circle A1301 centre (46.27, -45.16) radius 0.625
  circle A1302 centre (48.81, -45.16) radius 0.625
  circle A1303 centre (51.35, -45.16) radius 0.625
  circle A1304 centre (53.89, -45.16) radius 0.625
  circle A1305 centre (56.43, -45.16) radius 0.625
  circle A1306 centre (58.97, -45.16) radius 0.625
  circle A1307 centre (61.51, -45.16) radius 0.625
  circle A1308 centre (64.05, -45.16) radius 0.625
  circle A1309 centre (66.59, -45.16) radius 0.625
  circle A1310 centre (69.13, -45.16) radius 0.625
  circle A1311 centre (71.67, -45.16) radius 0.625
  circle A1312 centre (74.21, -45.16) radius 0.625
  circle A1313 centre (76.75, -45.16) radius 0.625
  circle A1314 centre (79.29, -45.16) radius 0.625
  circle A1315 centre (81.83, -45.16) radius 0.625
  circle A1316 centre (8.17, -47.7) radius 0.625
  circle A1317 centre (10.71, -47.7) radius 0.625
  circle A1318 centre (13.25, -47.7) radius 0.625
  circle A1319 centre (15.79, -47.7) radius 0.625
  circle A1320 centre (18.33, -47.7) radius 0.625
  circle A1321 centre (20.87, -47.7) radius 0.625
  circle A1322 centre (23.41, -47.7) radius 0.625
  circle A1323 centre (25.95, -47.7) radius 0.625
  circle A1324 centre (28.49, -47.7) radius 0.625
  circle A1325 centre (31.03, -47.7) radius 0.625
  circle A1326 centre (33.57, -47.7) radius 0.625
  circle A1327 centre (36.11, -47.7) radius 0.625
  circle A1328 centre (38.65, -47.7) radius 0.625
  circle A1329 centre (41.19, -47.7) radius 0.625
  circle A1330 centre (43.73, -47.7) radius 0.625
  circle A1331 centre (46.27, -47.7) radius 0.625
  circle A1332 centre (48.81, -47.7) radius 0.625
  circle A1333 centre (51.35, -47.7) radius 0.625
  circle A1334 centre (53.89, -47.7) radius 0.625
  circle A1335 centre (56.43, -47.7) radius 0.625
  circle A1336 centre (58.97, -47.7) radius 0.625
  circle A1337 centre (61.51, -47.7) radius 0.625
  circle A1338 centre (64.05, -47.7) radius 0.625
  circle A1339 centre (66.59, -47.7) radius 0.625
  circle A1340 centre (69.13, -47.7) radius 0.625
  circle A1341 centre (71.67, -47.7) radius 0.625
  circle A1342 centre (74.21, -47.7) radius 0.625
  circle A1343 centre (76.75, -47.7) radius 0.625
  circle A1344 centre (79.29, -47.7) radius 0.625
  circle A1345 centre (81.83, -47.7) radius 0.625
  circle A1346 centre (8.17, -50.24) radius 0.625
  circle A1347 centre (10.71, -50.24) radius 0.625
  circle A1348 centre (13.25, -50.24) radius 0.625
  circle A1349 centre (15.79, -50.24) radius 0.625
  circle A1350 centre (18.33, -50.24) radius 0.625
  circle A1351 centre (20.87, -50.24) radius 0.625
  circle A1352 centre (23.41, -50.24) radius 0.625
  circle A1353 centre (25.95, -50.24) radius 0.625
  circle A1354 centre (28.49, -50.24) radius 0.625
  circle A1355 centre (31.03, -50.24) radius 0.625
  circle A1356 centre (33.57, -50.24) radius 0.625
  circle A1357 centre (36.11, -50.24) radius 0.625
  circle A1358 centre (38.65, -50.24) radius 0.625
  circle A1359 centre (41.19, -50.24) radius 0.625
  circle A1360 centre (43.73, -50.24) radius 0.625
  circle A1361 centre (46.27, -50.24) radius 0.625
  circle A1362 centre (48.81, -50.24) radius 0.625
  circle A1363 centre (51.35, -50.24) radius 0.625
  circle A1364 centre (53.89, -50.24) radius 0.625
  circle A1365 centre (56.43, -50.24) radius 0.625
  circle A1366 centre (58.97, -50.24) radius 0.625
  circle A1367 centre (61.51, -50.24) radius 0.625
  circle A1368 centre (64.05, -50.24) radius 0.625
  circle A1369 centre (66.59, -50.24) radius 0.625
  circle A1370 centre (69.13, -50.24) radius 0.625
  circle A1371 centre (71.67, -50.24) radius 0.625
  circle A1372 centre (74.21, -50.24) radius 0.625
  circle A1373 centre (76.75, -50.24) radius 0.625
  circle A1374 centre (79.29, -50.24) radius 0.625
  circle A1375 centre (81.83, -50.24) radius 0.625
  circle A1376 centre (8.17, -52.78) radius 0.625
  circle A1377 centre (10.71, -52.78) radius 0.625
  circle A1378 centre (13.25, -52.78) radius 0.625
  circle A1379 centre (15.79, -52.78) radius 0.625
  circle A1380 centre (18.33, -52.78) radius 0.625
  circle A1381 centre (20.87, -52.78) radius 0.625
  circle A1382 centre (23.41, -52.78) radius 0.625
  circle A1383 centre (25.95, -52.78) radius 0.625
  circle A1384 centre (28.49, -52.78) radius 0.625
  circle A1385 centre (31.03, -52.78) radius 0.625
  circle A1386 centre (33.57, -52.78) radius 0.625
  circle A1387 centre (36.11, -52.78) radius 0.625
  circle A1388 centre (38.65, -52.78) radius 0.625
  circle A1389 centre (41.19, -52.78) radius 0.625
  circle A1390 centre (43.73, -52.78) radius 0.625
  circle A1391 centre (46.27, -52.78) radius 0.625
  circle A1392 centre (48.81, -52.78) radius 0.625
  circle A1393 centre (51.35, -52.78) radius 0.625
  circle A1394 centre (53.89, -52.78) radius 0.625
  circle A1395 centre (56.43, -52.78) radius 0.625
  circle A1396 centre (58.97, -52.78) radius 0.625
  circle A1397 centre (61.51, -52.78) radius 0.625
  circle A1398 centre (64.05, -52.78) radius 0.625
  circle A1399 centre (66.59, -52.78) radius 0.625
  circle A1400 centre (69.13, -52.78) radius 0.625
  circle A1401 centre (71.67, -52.78) radius 0.625
  circle A1402 centre (74.21, -52.78) radius 0.625
  circle A1403 centre (76.75, -52.78) radius 0.625
  circle A1404 centre (79.29, -52.78) radius 0.625
  circle A1405 centre (81.83, -52.78) radius 0.625
  circle A1406 centre (8.17, -55.32) radius 0.625
  circle A1407 centre (10.71, -55.32) radius 0.625
  circle A1408 centre (13.25, -55.32) radius 0.625
  circle A1409 centre (15.79, -55.32) radius 0.625
  circle A1410 centre (18.33, -55.32) radius 0.625
  circle A1411 centre (20.87, -55.32) radius 0.625
  circle A1412 centre (23.41, -55.32) radius 0.625
  circle A1413 centre (25.95, -55.32) radius 0.625
  circle A1414 centre (28.49, -55.32) radius 0.625
  circle A1415 centre (31.03, -55.32) radius 0.625
  circle A1416 centre (33.57, -55.32) radius 0.625
  circle A1417 centre (36.11, -55.32) radius 0.625
  circle A1418 centre (38.65, -55.32) radius 0.625
  circle A1419 centre (41.19, -55.32) radius 0.625
  circle A1420 centre (43.73, -55.32) radius 0.625
  circle A1421 centre (46.27, -55.32) radius 0.625
  circle A1422 centre (48.81, -55.32) radius 0.625
  circle A1423 centre (51.35, -55.32) radius 0.625
  circle A1424 centre (53.89, -55.32) radius 0.625
  circle A1425 centre (56.43, -55.32) radius 0.625
  circle A1426 centre (58.97, -55.32) radius 0.625
  circle A1427 centre (61.51, -55.32) radius 0.625
  circle A1428 centre (64.05, -55.32) radius 0.625
  circle A1429 centre (66.59, -55.32) radius 0.625
  circle A1430 centre (69.13, -55.32) radius 0.625
  circle A1431 centre (71.67, -55.32) radius 0.625
  circle A1432 centre (74.21, -55.32) radius 0.625
  circle A1433 centre (76.75, -55.32) radius 0.625
  circle A1434 centre (79.29, -55.32) radius 0.625
  circle A1435 centre (81.83, -55.32) radius 0.625
  circle A1436 centre (8.17, -57.86) radius 0.625
  circle A1437 centre (10.71, -57.86) radius 0.625
  circle A1438 centre (13.25, -57.86) radius 0.625
  circle A1439 centre (15.79, -57.86) radius 0.625
  circle A1440 centre (18.33, -57.86) radius 0.625
  circle A1441 centre (20.87, -57.86) radius 0.625
  circle A1442 centre (23.41, -57.86) radius 0.625
  circle A1443 centre (25.95, -57.86) radius 0.625
  circle A1444 centre (28.49, -57.86) radius 0.625
  circle A1445 centre (31.03, -57.86) radius 0.625
  circle A1446 centre (33.57, -57.86) radius 0.625
  circle A1447 centre (36.11, -57.86) radius 0.625
  circle A1448 centre (38.65, -57.86) radius 0.625
  circle A1449 centre (41.19, -57.86) radius 0.625
  circle A1450 centre (43.73, -57.86) radius 0.625
  circle A1451 centre (46.27, -57.86) radius 0.625
  circle A1452 centre (48.81, -57.86) radius 0.625
  circle A1453 centre (51.35, -57.86) radius 0.625
  circle A1454 centre (53.89, -57.86) radius 0.625
  circle A1455 centre (56.43, -57.86) radius 0.625
  circle A1456 centre (58.97, -57.86) radius 0.625
  circle A1457 centre (61.51, -57.86) radius 0.625
  circle A1458 centre (64.05, -57.86) radius 0.625
  circle A1459 centre (66.59, -57.86) radius 0.625
  circle A1460 centre (69.13, -57.86) radius 0.625
  circle A1461 centre (71.67, -57.86) radius 0.625
  circle A1462 centre (74.21, -57.86) radius 0.625
  circle A1463 centre (76.75, -57.86) radius 0.625
  circle A1464 centre (79.29, -57.86) radius 0.625
  circle A1465 centre (81.83, -57.86) radius 0.625
  circle A1466 centre (8.17, -60.4) radius 0.625
  circle A1467 centre (10.71, -60.4) radius 0.625
  circle A1468 centre (13.25, -60.4) radius 0.625
  circle A1469 centre (15.79, -60.4) radius 0.625
  circle A1470 centre (18.33, -60.4) radius 0.625
  circle A1471 centre (20.87, -60.4) radius 0.625
  circle A1472 centre (23.41, -60.4) radius 0.625
  circle A1473 centre (25.95, -60.4) radius 0.625
  circle A1474 centre (28.49, -60.4) radius 0.625
  circle A1475 centre (31.03, -60.4) radius 0.625
  circle A1476 centre (33.57, -60.4) radius 0.625
  circle A1477 centre (36.11, -60.4) radius 0.625
  circle A1478 centre (38.65, -60.4) radius 0.625
  circle A1479 centre (41.19, -60.4) radius 0.625
  circle A1480 centre (43.73, -60.4) radius 0.625
  circle A1481 centre (46.27, -60.4) radius 0.625
  circle A1482 centre (48.81, -60.4) radius 0.625
  circle A1483 centre (51.35, -60.4) radius 0.625
  circle A1484 centre (53.89, -60.4) radius 0.625
  circle A1485 centre (56.43, -60.4) radius 0.625
  circle A1486 centre (58.97, -60.4) radius 0.625
  circle A1487 centre (61.51, -60.4) radius 0.625
  circle A1488 centre (64.05, -60.4) radius 0.625
  circle A1489 centre (66.59, -60.4) radius 0.625
  circle A1490 centre (69.13, -60.4) radius 0.625
  circle A1491 centre (71.67, -60.4) radius 0.625
  circle A1492 centre (74.21, -60.4) radius 0.625
  circle A1493 centre (76.75, -60.4) radius 0.625
  circle A1494 centre (79.29, -60.4) radius 0.625
  circle A1495 centre (81.83, -60.4) radius 0.625